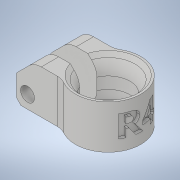
# Autodesk Inventor part: MINI-fan-spacer-clip
Saved by Autodesk Inventor 2021 (Build 250183000, 183)
## iProperties
Company: Prusa Development a.s.
RuleStatus: InUse
Created: 2019-12-20
Material: Všeobecné
Document SubType Name: Modeling
Designer: Alexandr Kukan
Density: 1 g/cm^3
Appearance: Výchozí
Project: ORIGINAL PRUSA MINI
Authority: Alexandr Kukan
Author: Alexandr Kukan
Title: MINI-fan-spacer-clip
Revision Number: R4
Autodesk Inventor part; units mm, degrees
ref_plane "XZ Plane" through (0, 0, 0) normal (0, 1, 0) x (-1, 0, 0)
ref_plane "XY Plane" through (0, 0, 0) normal (0, 0, 1) x (1, 0, 0)
sketch "Náčrt1" plane through (0, 0, 0) normal (0, 1, 0) x (-1, 0, 0)
  line L0 (0, -2) -> (0, 2)
  line L1 (0, 2) -> (24, 2)
  line L2 (24, 2) -> (24, -2)
  line L3 (24, -2) -> (0, -2)
  circle A0 centre (0, 0) radius 5
  circle A1 centre (0, 0) radius 7.5
  dimension "d0" = 4
  constraints: 8 end point, 3 perpendicular, 2 centre point, 2 coincident, 1 vertical
  measures "d0" distance of L0.start L0.end
sketch "Náčrt2" plane through (0, 0, 0) normal (0, 1, 0) x (-1, 0, 0)
  line L0 (4.5, 6) -> (17, 6)
  line L1 (17, 6) -> (18, 5)
  line L2 (18, 5) -> (18, -4.8205)
  line L3 (18, -4.8205) -> (17, -6)
  line L4 (17, -6) -> (4.5, -6)
  arc A0 (4.5, 6) -> (4.5, -6) centre (0, 0) ccw
  constraints: 10 end point, 2 point on circle, 1 centre point, 1 coincident, 1 horizontal, 1 parallel, 1 perpendicular
extrude "Vysunutí1" add sketch "Náčrt2" against normal blind 10
extrude "Vysunutí2" cut sketch "Náčrt1" against normal blind 10 contours L3 A0 L1 L0 | L0 L1 A0 L3 | A0 L1 A1 L3 | A1 L1 L2 L3 picked at (5.8076, -0.4525)
chamfer "Zkosení1" distance 2 angle 45 2 edges at (5, 0, 0) (5, -10, 0)
fillet "Zaoblení1" radius 4 2 edges at (5, -8, 0) (5, -2, 0)
sketch "Náčrt4" plane through (0, 0, 0) normal (0, 1, 0) x (1, 0, 0)
  line L0 (-15, 7) -> (-15, 6)
  line L1 (-17, 6) -> (-4.5, 6) projected
  line L2 (-16, 5) -> (-15, 6)
  line L3 (-16, 5) -> (-16, -5)
  line L4 (-16, -5) -> (-15, -6)
  line L5 (-15, -6) -> (-15, -7)
  line L6 (-15, -7) -> (-19, -7)
  line L7 (-19, -7) -> (-19, 7)
  line L8 (-19, 7) -> (-15, 7)
  point P0 (0, 0)
  constraints: 16 end point, 3 perpendicular, 2 point on line, 2 vertical
extrude "Vysunutí3" cut sketch "Náčrt4" against normal blind 10
sketch "Náčrt5" plane through (-4.5, -10, 6) normal (0, 0, 1) x (1, 0, 0)
  circle A0 centre (-8, 3) radius 1.6
  point P0 (4.5, 10)
  dimension "d12" = 3.2
  constraints: 1 centre point
  measures "d12" diameter of A0
extrude "Vysunutí4" cut sketch "Náčrt5" against normal blind 15
chamfer "Zkosení2" distance 2 angle 45 2 edges at (-16, -10, -3.5) (-16, -10, 3.5)
chamfer "Zkosení3" distance 5 angle 45 2 edges at (-16, 0, -3.5) (-16, 0, 3.5)
fillet "Zaoblení2" radius 4 6 edges at (-16, -5, -3.5) (-16, -8, -3.5) (-16, -8, 3.5) (-16, -5, 3.5) (-11, 0, -4) (-11, 0, 4)
fillet "Zaoblení3" radius 4 2 edges at (-4.5, -5, 6) (-4.5, -5, -6)
ref_plane "Pracovní rovina1" through (7.5, 0, 0) normal (1, 0, 0) x (0, 1, 0)
sketch "Náčrt7" plane through (7.5, 0, 0) normal (1, 0, 0) x (0, 1, 0)
  line L0 (0, -10.5) -> (0, 10.5) projected
  line L1 (-12, 0) -> (2, 0) projected
  line L2 (-10, 7.5) -> (-10, -7.5) projected
  line L3 (0.0851, 3.4066) -> (0.0851, -3.4066) construction
  line L4 (0.0851, -3.4066) -> (-10.0851, -3.4066) construction
  line L5 (-10.0851, -3.4066) -> (-10.0851, 3.4066) construction
  line L6 (-10.0851, 3.4066) -> (0.0851, 3.4066) construction
  line L7 (-7.4939, -0.4518) -> (-7.4939, 1.0758)
  line L8 (-7.4939, 1.0758) -> (-5.6584, 2.4656)
  line L9 (-5.6584, 2.4656) -> (-5.6584, 2.9194)
  line L10 (-5.6584, 2.9194) -> (-7.4939, 2.9194)
  line L11 (-7.4939, 2.9194) -> (-7.4939, 4.1673)
  line L12 (-7.4939, 4.1673) -> (-2.4939, 4.1673)
  line L13 (-2.4939, 4.1673) -> (-2.4939, 2.1576)
  spline S0 degree 2 poles (-2.4939, 2.1576) (-2.4939, 1.7403) (-2.5993, 1.1244) (-2.7613, 0.861) knots 0 0 0 1 2 2 2
  spline S1 degree 2 poles (-2.7613, 0.861) (-2.9315, 0.5936) (-3.4623, 0.2776) (-3.8675, 0.2776) knots 0 0 0 1 2 2 2
  spline S2 degree 2 poles (-3.8675, 0.2776) (-4.4388, 0.2776) (-5.156, 0.7962) (-5.3667, 1.2297) knots 0 0 0 1 2 2 2
  line L14 (-5.3667, 1.2297) -> (-7.4939, -0.4518)
  spline S3 degree 2 poles (-4.0255, 1.566) (-3.8351, 1.566) (-3.5636, 1.7119) (-3.4907, 1.878) knots 0 0 0 1 2 2 2
  spline S4 degree 2 poles (-3.4907, 1.878) (-3.4421, 1.9955) (-3.4137, 2.2832) (-3.4137, 2.498) knots 0 0 0 1 2 2 2
  line L15 (-3.4137, 2.498) -> (-3.4137, 2.9194)
  line L16 (-3.4137, 2.9194) -> (-4.7589, 2.9194)
  line L17 (-4.7589, 2.9194) -> (-4.7589, 2.5588)
  spline S5 degree 2 poles (-4.7589, 2.5588) (-4.7589, 2.2994) (-4.6941, 1.9307) (-4.5928, 1.8051) knots 0 0 0 1 2 2 2
  spline S6 degree 2 poles (-4.5928, 1.8051) (-4.4955, 1.6835) (-4.2362, 1.566) (-4.0255, 1.566) knots 0 0 0 1 2 2 2
  line L18 (-6.327, -4.5482) -> (-6.327, -3.8716)
  line L19 (-6.327, -3.8716) -> (-7.5061, -3.8716)
  line L20 (-7.5061, -3.8716) -> (-7.5061, -2.66)
  line L21 (-7.5061, -2.66) -> (-6.327, -2.66)
  line L22 (-6.327, -2.66) -> (-6.327, -0.4558)
  line L23 (-6.327, -0.4558) -> (-5.3951, -0.4558)
  line L24 (-5.3951, -0.4558) -> (-2.4939, -2.6195)
  line L25 (-2.4939, -2.6195) -> (-2.4939, -3.8716)
  line L26 (-2.4939, -3.8716) -> (-5.4275, -3.8716)
  line L27 (-5.4275, -3.8716) -> (-5.4275, -4.5482)
  line L28 (-5.4275, -4.5482) -> (-6.327, -4.5482)
  line L29 (-5.4275, -2.66) -> (-3.7257, -2.66)
  line L30 (-3.7257, -2.66) -> (-5.4275, -1.3918)
  line L31 (-5.4275, -1.3918) -> (-5.4275, -2.66)
  point P0 (0, 0)
  point P1 (-10, -6.5217)
  point P2 (-10, 6.5217)
  point P3 (-5, 3.4066)
  point P4 (0.0851, 0)
  dimension "rev_num" = 4
  dimension "d23" = 5
  constraints: 2 midpoint, 1 point on line, 2 other
  measures "d23" distance from line of L0 point (-5, 3.407)
emboss "Reliéf1" sketch "Náčrt7" operation cut depth 0.7 direction (1, 0, 0) wrap yes faces at (7.4937, -6.6667, -0.3069)
equation "\"rev_num\" = 4"
equation "\"d23\" = 0.5 * d2"
equation "\"d2\" = 10"
